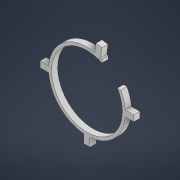
# Autodesk Inventor part: Clip_TestFitV1
Saved by Autodesk Inventor 2022 (Build 260153000, 153)
## iProperties
Created: 2023-05-05
Part Number: Clip_TestFitV1
Material: Generic
Document SubType Name: Modeling
Designer: User
Density: 1 g/cm^3
Appearance: Default
Author: User
Autodesk Inventor part; units mm, degrees
ref_plane "YZ Plane" through (0, 0, 0) normal (1, 0, 0) x (0, 1, 0)
ref_plane "XZ Plane" through (0, 0, 0) normal (0, 1, 0) x (-1, 0, 0)
ref_plane "XY Plane" through (0, 0, 0) normal (0, 0, 1) x (1, 0, 0)
sketch "Sketch1" plane through (0, 0, 0) normal (0, 0, 1) x (1, 0, 0)
  arc A0 (-25.4018, 15) -> (25.4018, 15) centre (0, 0) ccw
  line L0 (25.4018, 15) -> (28.2666, 15)
  line L1 (-39, 2.5) -> (-32, 2.5)
  line L2 (-32, -2.5) -> (-39, -2.5)
  line L3 (-39, -2.5) -> (-39, 2.5)
  line L4 (-32, 2.5) -> (-31.9022, 2.5)
  line L5 (-32, -2.5) -> (-31.9022, -2.5)
  line L6 (2.5, -32) -> (2.5, -39)
  line L7 (2.5, -39) -> (-2.5, -39)
  line L8 (-2.5, -39) -> (-2.5, -32)
  line L9 (-2.5, -32) -> (-2.5, -31.9022)
  line L10 (2.5, -32) -> (2.5, -31.9022)
  line L11 (32, 2.5) -> (39, 2.5)
  line L12 (39, 2.5) -> (39, -2.5)
  line L13 (39, -2.5) -> (32, -2.5)
  line L14 (32, 2.5) -> (31.9022, 2.5)
  line L15 (32, -2.5) -> (31.9022, -2.5)
  arc A1 (-28.2666, 15) -> (-31.9022, 2.5) centre (0, 0) ccw
  arc A2 (-31.9022, -2.5) -> (-2.5, -31.9022) centre (0, 0) ccw
  arc A3 (2.5, -31.9022) -> (31.9022, -2.5) centre (0, 0) ccw
  arc A4 (31.9022, 2.5) -> (28.2666, 15) centre (0, 0) ccw
  arc A5 (12.5, 26.7208) -> (25.4018, 15) centre (0, 0) ccw
  line L16 (12.5, 29.4576) -> (12.5, 26.7208)
  arc A6 (-2.5, 31.9022) -> (-31.9022, 2.5) centre (0, 0) ccw
  arc A7 (-31.9022, -2.5) -> (-2.5, -31.9022) centre (0, 0) ccw
  arc A8 (2.5, -31.9022) -> (31.9022, -2.5) centre (0, 0) ccw
  arc A9 (31.9022, 2.5) -> (28.2666, 15) centre (0, 0) ccw
  line L17 (6.5, 31.3329) -> (7.5001, 38.3601)
  line L18 (6.5, 31.3329) -> (13.598, 31.3329) construction
  line L19 (7.5001, 38.3601) -> (12.4502, 37.6556)
  line L20 (12.4502, 37.6556) -> (11.3493, 29.9198)
  arc A10 (12.5, 29.4576) -> (11.3493, 29.9198) centre (0, 0) ccw
  arc A11 (12.5, 29.4576) -> (11.3493, 29.9198) centre (0, 0) ccw
  arc A12 (6.5, 31.3329) -> (2.5, 31.9022) centre (0, 0) ccw
  arc A13 (6.5, 31.3329) -> (-31.9022, 2.5) centre (0, 0) ccw
  arc A14 (31.9022, 2.5) -> (28.2666, 15) centre (0, 0) ccw
  arc A15 (-31.9022, -2.5) -> (-2.5, -31.9022) centre (0, 0) ccw
  arc A16 (2.5, -31.9022) -> (31.9022, -2.5) centre (0, 0) ccw
  point P0 (11.5, 29.8622)
  point P1 (2.5, 31.9022)
  dimension "d78" = 7.098
  dimension "d79" = 81.9
  dimension "d80" = 5
  dimension "d81" = 90
  dimension "d82" = 90
  constraints: 42 end point, 35 point on circle, 17 centre point, 7 horizontal, 5 coincident, 3 parallel, 2 perpendicular, 2 vertical, 1 equal length
  measures "d78" distance of L17.start L17.end
  measures "d79" angle of L18 L17
  measures "d80" distance of L17.end L19.end
  measures "d81" angle of L17 L19
  measures "d82" angle of L19 L20
extrude "Extrusion6" add sketch "Sketch1" along normal blind 5
body "Solid4"
